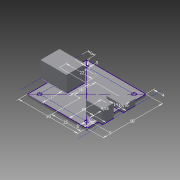
# Autodesk Inventor part: PCB-Model
Saved by Autodesk Inventor 2014 (Build 180170000, 170)
## iProperties
Created: 2013-01-07
Part Number: PCB-Model
Material: Generic
Document SubType Name: Modeling
Designer: md
Density: 1 g/cm^3
Appearance: Default
Author: md
Autodesk Inventor part; units mm, degrees
ref_plane "YZ Plane" through (0, 0, 0) normal (1, 0, 0) x (0, 1, 0)
ref_plane "XZ Plane" through (0, 0, 0) normal (0, 1, 0) x (-1, 0, 0)
ref_plane "XY Plane" through (0, 0, 0) normal (0, 0, 1) x (1, 0, 0)
sketch "Platine" plane through (0, 0, 0) normal (0, 0, 1) x (1, 0, 0)
  line L0 (-25, -19.16) -> (25, -19.16)
  line L1 (25, -19.16) -> (25, 30.84)
  line L2 (25, 30.84) -> (-25, 30.84)
  line L3 (-25, 30.84) -> (-25, -19.16)
  line L4 (-25, -19.16) -> (25, 30.84)
  line L5 (25, -19.16) -> (-25, 30.84)
  line L6 (-31, -2.16) -> (-9, -2.16)
  line L7 (-9, -2.16) -> (-9, 13.84)
  line L8 (-9, 13.84) -> (-31, 13.84)
  line L9 (-31, 13.84) -> (-31, -2.16)
  line L10 (29, -9.76) -> (15, -9.76)
  line L11 (15, -9.76) -> (15, -0.21)
  line L12 (15, -0.21) -> (29, -0.21)
  line L13 (29, -0.21) -> (29, -9.76)
  line L14 (15, 7.84) -> (29, 7.84)
  line L15 (29, 7.84) -> (29, 18)
  line L16 (29, 18) -> (15, 18)
  line L17 (15, 18) -> (15, 7.84)
  circle A0 centre (-20, 25.84) radius 1.5
  circle A1 centre (20, -14.16) radius 1.5
  line L18 (-31, 32.4529) -> (-31, -19) construction
  line L19 (29, 40.2658) -> (29, -31.3692) construction
  line L20 (-20, 25.84) -> (20, 25.84) construction
  line L21 (20, 25.84) -> (20, -14.16) construction
  line L22 (20, -14.16) -> (-20, -14.16) construction
  line L23 (-20, -14.16) -> (-20, 25.84) construction
  circle A2 centre (20, 25.84) radius 1.5
  circle A3 centre (-20, -14.16) radius 1.5
  point P0 (0, 0)
  point P1 (0, 5.84)
  dimension "d0" = 50
  dimension "d1" = 50
  dimension "d2" = 22
  dimension "d3" = 16
  dimension "d4" = 17
  dimension "d6" = 14
  dimension "d7" = 9.55
  dimension "d8" = 9.4
  dimension "d10" = 10.16
  dimension "d11" = 14
  dimension "d12" = 27
  dimension "d14" = 3
  dimension "d15" = 5
  dimension "d16" = 5
  dimension "d17" = 5
  dimension "d18" = 5
  dimension "d19" = 18
  dimension "d127" = 6
  dimension "d128" = 4
  dimension "d129" = 25
  constraints: 48 end point, 12 parallel, 5 horizontal, 5 perpendicular, 4 centre point, 3 collinear, 3 equal radius, 2 coincident, 2 midpoint
  measures "d0" distance between parallel lines of L0 L2
  measures "d1" distance between parallel lines of L1 L3
  measures "d2" distance between parallel lines of L7 L9
  measures "d3" distance of L8.end L6.start
  measures "d4" distance between parallel lines of L6 L0
  measures "d6" distance between parallel lines of L13 L11
  measures "d7" distance between parallel lines of L10 L12
  measures "d8" distance between parallel lines of L0 L10
  measures "d10" distance between parallel lines of L14 L16
  measures "d11" distance between parallel lines of L15 L17
  measures "d12" distance between parallel lines of L0 L14
  measures "d14" diameter of A0
  measures "d15" distance from line of L20.start L3
  measures "d16" distance from line of L20.start L2
  measures "d17" distance from line of L21.end L1
  measures "d18" distance from line of L21.end L0
  measures "d19" distance from line of point (0, 0) L16
  measures "d127" distance between parallel lines of L3 L18
  measures "d128" distance between parallel lines of L19 L1
  measures "d129" distance from line of L1 point (0, 0)
extrude "Platinengeometrie" add sketch "Platine" against normal blind 2 contours L4 A3 L5 L11 L10 A1 L0 | L3 L6 L7 L8 L5 A0 L4 A3 | L5 A1 L10 L1 | L3 L8 L7 L6 | A3 L4 | L4 A3 | L10 L5 L11 L12 L1 | A1 L5 | L5 A1 | L12 L11 L5 L4 A2 L1 L16 L17 L14 | L10 L11 L5 | L2 L4 A2 L5 A0 | L14 L17 L16 L1 | A0 L5 | L5 A0 | A2 L4 | L4 A2
extrude "MEBP 8-8G" add sketch "Platine" along normal blind 13.5 contours L6 L9 L8 L3 | L3 L8 L7 L6
extrude "HEBW21" add sketch "Platine" along normal blind 11 contours L10 L5 L11 L12 L1 | L1 L12 L13 L10 | L10 L11 L5
extrude "PSS 254/4W" add sketch "Platine" along normal blind 5 contours L14 L17 L16 L1 | L1 L16 L15 L14
extrude "Extrusion9" cut sketch "Platine" against normal up to next contours A1 L5 | L5 A1 | A0 L5 | L5 A0
equation "\"d136\" = d18"
